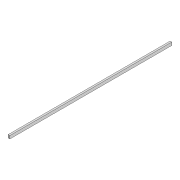
# Autodesk Inventor part: batang
Saved by Autodesk Inventor 2020 (Build 240168000, 168)
## iProperties
Created: 2020-03-24
Part Number: batang
Material: Generic
Document SubType Name: Modeling
Designer: alifhabib
Density: 1 g/cm^3
Appearance: Default
Author: alifhabib
Autodesk Inventor part; units mm, degrees
ref_plane "YZ Plane" through (0, 0, 0) normal (1, 0, 0) x (0, 1, 0)
ref_plane "XZ Plane" through (0, 0, 0) normal (0, 1, 0) x (-1, 0, 0)
ref_plane "XY Plane" through (0, 0, 0) normal (0, 0, 1) x (1, 0, 0)
sketch "Sketch1" plane through (0, 0, 0) normal (0, 0, 1) x (1, 0, 0)
  line L0 (-5.95, 9.95) -> (5.95, 9.95)
  line L1 (5.95, 9.95) -> (5.95, -9.95)
  line L2 (5.95, -9.95) -> (-5.95, -9.95)
  line L3 (-5.95, -9.95) -> (-5.95, 9.95)
  line L4 (-5.95, 9.95) -> (5.95, -9.95) construction
  line L5 (5.95, 9.95) -> (-5.95, -9.95) construction
  point P0 (0, 0)
  dimension "d0" = 11.9
  dimension "d1" = 19.9
  constraints: 12 end point, 2 midpoint, 2 parallel, 1 horizontal, 1 perpendicular
  measures "d0" distance of L1.end L2.end
  measures "d1" distance of L0.end L1.end
extrude "Extrusion1" add sketch "Sketch1" along normal blind 1100
body "Solid1"
